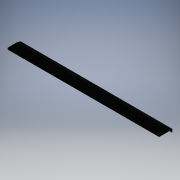
# Autodesk Inventor part: Blackside
Saved by Autodesk Inventor 2016 (Build 200138000, 138)
## iProperties
Created: 2015-05-19
Part Number: Blackside
Material: Steel
Document SubType Name: Modeling
Designer: Andy
Density: 7.85 g/cm^3
Appearance: Plate
Mass: 3120.53 g
Surface Area: 1357.72 cm^2
Volume: 397.52 cm^3
Author: Andy
Autodesk Inventor part; units mm, degrees
ref_plane "YZ Plane" through (0, 0, 0) normal (1, 0, 0) x (0, 1, 0)
ref_plane "XZ Plane" through (0, 0, 0) normal (0, 1, 0) x (-1, 0, 0)
ref_plane "XY Plane" through (0, 0, 0) normal (0, 0, 1) x (1, 0, 0)
sketch "Sketch1" plane through (0, 0, 0) normal (1, 0, 0) x (0, 1, 0)
  line L0 (10, 0) -> (58, 0)
  line L1 (78, -10) -> (78, -21)
  line L2 (78, -21) -> (78, -10)
  line L3 (78, -21) -> (78, -10)
  line L4 (78, -10) -> (78, -21)
  line L5 (58, 0) -> (10, 0)
  line L6 (58, 0) -> (10, 0)
  line L7 (78, -21) -> (78, -6)
  line L8 (78, -6) -> (58, 0)
  line L9 (78, -21) -> (76, -21)
  line L10 (76, -21) -> (76, -8)
  line L11 (10, -8) -> (76, -8)
  line L12 (10, -8) -> (10, 0)
  point P0 (0, 0)
  dimension "d6" = 15
  dimension "d9" = 2
  constraints: 26 end point, 4 perpendicular, 1 collinear, 1 horizontal, 1 point on line
  measures "d6" distance of L1.end L7.end
  measures "d9" distance of L1.end L9.end
extrude "Extrusion1" add sketch "Sketch1" along normal blind 779.45
body "Solid1"
